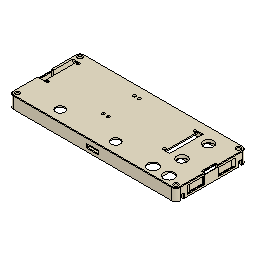
Font Plates (Autodesk Fusion 360 design; units mm, degrees)
Autodesk Fusion 360 part; units mm, degrees
sketch "Sketch1" plane through (0, 0, 0) normal (0, 0, 1) x (1, 0, 0)
  line L0 (0, 0) -> (200, 0)
  line L1 (200, 0) -> (200, 85)
  line L2 (200, 85) -> (0, 85)
  line L3 (0, 85) -> (0, 0)
  dimension "d1" = 200
  dimension "d2" = 85
  constraint horizontal L0
  constraint vertical L1
  constraint horizontal L2
  constraint vertical L3
  constraint coincident L0.start L3.end
  measures "d1" distance of L0.start L0.end
  measures "d2" distance of L0.start L2.end
extrude "Extrude1" add sketch "Sketch1" along normal blind 1.5 makes body 1
sketch "Sketch2" plane through (0, 0, 1.5) normal (0, 0, 1) x (-1, 0, 0)
  line L0 (0, -85) -> (0, 0)
  line L1 (0, 0) -> (-200, 0)
  line L2 (-200, 0) -> (-200, -85)
  line L3 (-200, -85) -> (0, -85)
  line L4 (-100, -85) -> (-100, 0) construction
  line L5 (0, -42.5) -> (-200, -42.5) construction
  line L6 (-3, -3) -> (-197, -3)
  line L7 (-197, -3) -> (-197, -82)
  line L8 (-197, -82) -> (-3, -82)
  line L9 (-3, -82) -> (-3, -3)
  dimension "d176" = -3
  constraint midpoint L1 L4.end
  constraint midpoint L0 L5.start
  constraint midpoint L3 L4.start
  constraint midpoint L2 L5.end
extrude "Extrude2" add sketch "Sketch2" along normal blind 13.7 bodies 1
sketch "Sketch4" plane through (197, 0, 0) normal (-1, 0, 0) x (0, -1, 0)
  line L0 (-50.25, 1.5) -> (-34.75, 1.5)
  line L1 (-34.75, 1.5) -> (-34.75, 9.1)
  line L2 (-34.75, 9.1) -> (-50.25, 9.1)
  line L3 (-50.25, 9.1) -> (-50.25, 1.5)
  line L4 (-42.5, 15.2) -> (-42.5, 1.5) construction
  line L5 (-82, 1.5) -> (-3, 1.5)
  line L6 (-3, 1.5) -> (-3, 15.2)
  line L7 (-3, 15.2) -> (-82, 15.2)
  line L8 (-82, 15.2) -> (-82, 1.5)
  dimension "d84" = 15.5
  dimension "d284" = 7.6
  constraint horizontal L0
  constraint vertical L1
  constraint horizontal L2
  constraint vertical L3
  constraint midpoint L0 L4.end
  constraint perpendicular L0 L4
  constraint coincident L4.end L5
  constraint midpoint L4.start L7
  measures "d84" distance of L1 L3
  measures "d284" distance of L0.end L1.end
extrude "Extrude4" cut sketch "Sketch4" against normal blind 1.85 contours L0 L1 L2 L3 L5 bodies 1
ref_plane "WorkPlane3" through (100, 42.5, 7.6) normal (-1, 0, 0) x (0, -1, 0)
mirror "Mirror1" about plane through (100, 42.5, 7.6) normal (-1, 0, 0) of "Extrude4"
sketch "Sketch6" plane through (0, 82, 0) normal (0, -1, 0) x (1, 0, 0)
  line L0 (93.5, 10.1) -> (106.5, 10.1)
  line L1 (106.5, 10.1) -> (106.5, 6.6)
  line L2 (106.5, 6.6) -> (93.5, 6.6)
  line L3 (93.5, 6.6) -> (93.5, 10.1)
  line L4 (100, 15.2) -> (100, 1.5) construction
  line L5 (100, 10.1) -> (100, 6.6) construction
  circle A0 centre (169, 8.35) radius 2
  line L6 (169, 15.2) -> (169, 1.5) construction
  circle A1 centre (31, 8.35) radius 2
  line L7 (3, 1.5) -> (197, 1.5)
  line L8 (197, 1.5) -> (197, 15.2)
  line L9 (197, 15.2) -> (3, 15.2)
  line L10 (3, 15.2) -> (3, 1.5)
  dimension "d25" = 13
  dimension "d26" = 3.5
  dimension "d27" = 4
  dimension "d179" = 28
  constraint horizontal L0
  constraint vertical L1
  constraint horizontal L2
  constraint vertical L3
  constraint midpoint L0 L5.start
  constraint midpoint L2 L5.end
  constraint midpoint L4 L5
  constraint midpoint A0.centre L6
  constraint symmetric L4 A0 A1
  constraint coincident L4.start L9
  constraint midpoint L4.start L9
  constraint midpoint L4.end L7
  constraint coincident L6.start L9
  constraint coincident L6.end L7
  measures "d25" distance of L0.start L0.end
  measures "d26" distance of L0.start L2.end
  measures "d27" diameter of A0
  measures "d179" distance of L6 L8
extrude "Extrude7" cut sketch "Sketch6" against normal through all and the other way through all contours L0 L1 L2 L3 bodies 1
sketch "Sketch3" plane through (0, 0, 0) normal (0, 0, -1) x (1, 0, 0)
  line L0 (0, 0) -> (0, -85)
  line L1 (0, -85) -> (200, -85)
  line L2 (200, -85) -> (200, 0)
  line L3 (200, 0) -> (0, 0)
  line L4 (200, -50.25) -> (197, -50.25)
  line L5 (197, -50.25) -> (197, -34.75)
  line L6 (197, -34.75) -> (200, -34.75)
  line L7 (200, -34.75) -> (200, -50.25)
  line L8 (100, -85) -> (100, 0) construction
  line L9 (3, -50.25) -> (3, -34.75)
  line L10 (3, -34.75) -> (0, -34.75)
  line L11 (0, -34.75) -> (0, -50.25)
  line L12 (0, -50.25) -> (3, -50.25)
  dimension "d11" = 3
  dimension "d12" = 15.5
  constraint horizontal L4
  constraint vertical L5
  constraint horizontal L6
  constraint vertical L7
  constraint coincident L2 L4.start
  constraint midpoint L2 L7
  constraint midpoint L1 L8.start
  constraint midpoint L3 L8.end
  constraint symmetric L4.start L8 L11.end
  constraint symmetric L4.end L8 L9.start
  constraint symmetric L5.end L8 L9.end
  constraint symmetric L6.end L8 L10.end
  measures "d11" distance of L4.start L4.end
  measures "d12" distance of L4.end L5.end
extrude "Extrude3" cut sketch "Sketch3" against normal blind 2.1 contours L0 L9 L10 L11 L12 | L2 L4 L5 L6 L7 bodies 1
sketch "Sketch25" plane through (200, 0, 0) normal (1, 0, 0) x (0, 1, 0)
  line L0 (34.75, 0) -> (34.75, 2.1)
  line L1 (34.75, 2.1) -> (50.25, 2.1)
  line L2 (50.25, 2.1) -> (50.25, 0)
  line L3 (50.25, 0) -> (85, 0)
  line L4 (85, 0) -> (85, 15.2)
  line L5 (85, 15.2) -> (0, 15.2)
  line L6 (0, 15.2) -> (0, 0)
  line L7 (0, 0) -> (34.75, 0)
  line L8 (42.5, 15.2) -> (42.5, 0) construction
  line L9 (78.9, 15.2) -> (75.9, 15.2)
  line L10 (75.9, 15.2) -> (75.9, 9.2)
  line L11 (75.9, 9.2) -> (78.9, 9.2)
  line L12 (78.9, 9.2) -> (78.9, 15.2)
  line L13 (77.4, 9.2) -> (77.4, 15.2) construction
  line L14 (9.1, 15.2) -> (9.1, 9.2)
  line L15 (9.1, 9.2) -> (6.1, 9.2)
  line L16 (6.1, 9.2) -> (6.1, 15.2)
  dimension "d248" = 3
  dimension "d249" = 6
  dimension "d250" = 34.9
  constraint midpoint L5 L8.start
  constraint perpendicular L5 L8
  constraint horizontal L9
  constraint vertical L10
  constraint horizontal L11
  constraint vertical L12
  constraint coincident L5 L9.start
  constraint midpoint L11 L13.start
  constraint midpoint L9 L13.end
  constraint symmetric L8 L9.start L16.end
  constraint symmetric L8 L9.end L14.start
  constraint symmetric L8 L10.end L14.end
  constraint symmetric L8 L11.end L15.end
  measures "d248" distance of L9.start L9.end
  measures "d249" distance of L9.start L11.end
  measures "d250" distance of L8 L13
extrude "Extrude28" cut sketch "Sketch25" against normal up to surface (3 mm away) contours L5 L14 L15 L16 | L5 L9 L10 L11 L12 bodies 1
sketch "Sketch26" plane through (200, 0, 0) normal (1, 0, 0) x (0, 1, 0)
  line L0 (78.9, 15.2) -> (78.9, 9.2)
  line L1 (78.9, 9.2) -> (75.9, 9.2)
  line L2 (75.9, 9.2) -> (75.9, 15.2)
  line L3 (75.9, 15.2) -> (9.1, 15.2)
  line L4 (9.1, 15.2) -> (9.1, 9.2)
  line L5 (9.1, 9.2) -> (6.1, 9.2)
  line L6 (6.1, 9.2) -> (6.1, 15.2)
  line L7 (6.1, 15.2) -> (0, 15.2)
  line L8 (0, 15.2) -> (0, 0)
  line L9 (0, 0) -> (34.75, 0)
  line L10 (34.75, 0) -> (34.75, 2.1)
  line L11 (34.75, 2.1) -> (50.25, 2.1)
  line L12 (50.25, 2.1) -> (50.25, 0)
  line L13 (50.25, 0) -> (85, 0)
  line L14 (85, 0) -> (85, 15.2)
  line L15 (85, 15.2) -> (78.9, 15.2)
  line L16 (67.5, 3.5) -> (51.5, 3.5)
  line L17 (51.5, 3.5) -> (51.5, 11.5)
  line L18 (51.5, 11.5) -> (67.5, 11.5)
  line L19 (67.5, 11.5) -> (67.5, 3.5)
  line L20 (67.5, 7.5) -> (51.5, 7.5) construction
  dimension "d253" = 16
  dimension "d254" = 8
  dimension "d255" = 17.5
  dimension "d256" = 7.5
  constraint horizontal L16
  constraint vertical L17
  constraint horizontal L18
  constraint vertical L19
  constraint midpoint L19 L20.start
  constraint midpoint L17 L20.end
  measures "d253" distance of L16.start L16.end
  measures "d254" distance of L16.start L18.end
  measures "d255" distance of L14 L19
  measures "d256" distance of L13 L20
extrude "Extrude29" cut sketch "Sketch26" against normal blind 1.5 contours L16 L17 L18 L19 bodies 1
sketch "Sketch28" plane through (0, 0, 3.5) normal (0, 0, 1) x (-1, 0, 0)
  line L0 (-200, -51.5) -> (-200, -67.5)
  line L1 (-200, -67.5) -> (-198.5, -67.5)
  line L2 (-198.5, -67.5) -> (-198.5, -51.5)
  line L3 (-198.5, -51.5) -> (-200, -51.5)
  line L4 (-200, -50.25) -> (-200, -85)
  line L5 (-198.5, -67.5) -> (-200, -71.1213)
  line L6 (-198.5, -67.5) -> (-194.5803, -67.5) construction
  dimension "d268" = 112.5
  constraint horizontal L6
  constraint coincident L1.end L2.start
  constraint coincident L4 L5.end
  measures "d268" angle of L5 L6
extrude "Extrude31" cut sketch "Sketch28" along normal up to surface (8 mm away) contours L1 L4 L5 bodies 1
ref_plane "WorkPlane5" through (100, 42.5, 7.6) normal (0, -1, 0) x (1, 0, 0)
mirror "Mirror5" about plane through (100, 42.5, 7.6) normal (0, -1, 0) of "Extrude29", "Extrude31"
mirror "Mirror4" about plane through (100, 42.5, 7.6) normal (-1, 0, 0) of "Extrude28", "Extrude29", "Extrude31", "Mirror5"
fillet "Fillet10" radius 5 8 edges at (0, 85, 7.6) (0, 0, 7.6) (200, 0, 7.6) (200, 85, 7.6) (197, 3, 8.35) (3, 3, 8.35) (3, 82, 8.35) (197, 82, 8.35) on bodies 1
chamfer "Chamfer9" distance 0.8 angle 45 4 faces at (69.3333, 84, 15.2) (69.3333, 1, 15.2) (199, 31.3667, 15.2) (1, 53.6333, 15.2) on bodies 1
chamfer "Chamfer7" distance 0.6 angle 45 16 edges at (100, 85, 0) (198.5355, 83.5355, 0) (200, 65.125, 0) (0, 65.125, 0) (1.4645, 83.5355, 0) (0, 19.875, 0) (1.4645, 1.4645, 0) (100, 0, 0) (198.5355, 1.4645, 0) (200, 19.875, 0) (197, 42.5, 0) (198.5, 50.25, 0) (198.5, 34.75, 0) (1.5, 50.25, 0) (3, 42.5, 0) (1.5, 34.75, 0) on bodies 1
chamfer "Chamfer8" distance 0.6 angle 45 50 edges at (100, 85, 10.1) (93.5, 85, 8.35) (100, 85, 6.6) (106.5, 85, 8.35) (1.15, 42.5, 2.1) (100, 0, 10.1) (106.5, 0, 8.35) (100, 0, 6.6) (93.5, 0, 8.35) (198.85, 42.5, 2.1) (200, 78.9, 11.8) (200, 75.9, 11.8) (196.9053, 77.9683, 9.2) (197, 76.45, 9.2) (196.6249, 78.9, 11.8) (197, 75.9, 11.8) (200, 77.4, 9.2) (200, 9.1, 11.8) (200, 7.6, 9.2) (197, 8.55, 9.2) (196.9053, 7.0317, 9.2) (197, 9.1, 11.8) (200, 6.1, 11.8) (196.6249, 6.1, 11.8) (3.0947, 7.0317, 9.2) (3, 8.55, 9.2) (3.3751, 6.1, 11.8) (0, 9.1, 11.8) (0, 7.6, 9.2) (0, 6.1, 11.8) (3, 9.1, 11.8) (3.3751, 78.9, 11.8) (3.0947, 77.9683, 9.2) (3, 76.45, 9.2) (3, 75.9, 11.8) (0, 75.9, 11.8) (0, 77.4, 9.2) (0, 78.9, 11.8) (0, 61.3107, 3.5) (0, 61.3107, 11.5) (0, 51.5, 7.5) (200, 61.3107, 3.5) (200, 51.5, 7.5) (200, 61.3107, 11.5) (0, 23.6893, 3.5) (0, 33.5, 7.5) (0, 23.6893, 11.5) (200, 23.6893, 11.5) (200, 33.5, 7.5) (200, 23.6893, 3.5) on bodies 1
sketch "Sketch13" plane through (0, 0, 0) normal (0, 0, 1) x (1, 0, 0)
  line L0 (5, 85) -> (195, 85)
  arc A0 (5, 85) -> (0, 80) centre (5, 80) ccw
  line L1 (0, 50.25) -> (0, 80)
  line L2 (0, 50.25) -> (0, 34.75)
  line L3 (0, 5) -> (0, 34.75)
  arc A1 (0, 5) -> (5, 0) centre (5, 5) ccw
  line L4 (195, 0) -> (5, 0)
  arc A2 (195, 0) -> (200, 5) centre (195, 5) ccw
  line L5 (200, 34.75) -> (200, 5)
  line L6 (200, 34.75) -> (200, 50.25)
  line L7 (200, 80) -> (200, 50.25)
  arc A3 (200, 80) -> (195, 85) centre (195, 80) ccw
  line L8 (200.1, 34.75) -> (200.1, 50.25)
  line L9 (200.1, 80) -> (200.1, 50.25)
  arc A4 (200.1, 80) -> (195, 85.1) centre (195, 80) ccw
  line L10 (5, 85.1) -> (195, 85.1)
  arc A5 (5, 85.1) -> (-0.1, 80) centre (5, 80) ccw
  line L11 (-0.1, 50.25) -> (-0.1, 80)
  line L12 (-0.1, 50.25) -> (-0.1, 34.75)
  line L13 (-0.1, 5) -> (-0.1, 34.75)
  arc A6 (-0.1, 5) -> (5, -0.1) centre (5, 5) ccw
  line L14 (195, -0.1) -> (5, -0.1)
  arc A7 (195, -0.1) -> (200.1, 5) centre (195, 5) ccw
  line L15 (200.1, 34.75) -> (200.1, 5)
  line L16 (-2.5, 5) -> (-2.5, 34.75)
  line L17 (-2.5, 50.25) -> (-2.5, 34.75)
  line L18 (-2.5, 50.25) -> (-2.5, 80)
  arc A8 (5, 87.5) -> (-2.5, 80) centre (5, 80) ccw
  line L19 (5, 87.5) -> (195, 87.5)
  arc A9 (202.5, 80) -> (195, 87.5) centre (195, 80) ccw
  line L20 (202.5, 80) -> (202.5, 50.25)
  line L21 (202.5, 34.75) -> (202.5, 50.25)
  line L22 (202.5, 34.75) -> (202.5, 5)
  arc A10 (195, -2.5) -> (202.5, 5) centre (195, 5) ccw
  line L23 (195, -2.5) -> (5, -2.5)
  arc A11 (-2.5, 5) -> (5, -2.5) centre (5, 5) ccw
  dimension "d191" = 0.1
  dimension "d192" = 2.5
extrude "Extrude14" add sketch "Sketch13" along normal mid plane 15.6 separate body contours L16 L17 L18 A8 L19 A9 L20 L21 L22 A10 L23 A11 makes body 2
sketch "Sketch12" plane through (0, 0, 0) normal (0, 0, -1) x (1, 0, 0)
  line L0 (3, -11.5) -> (8.5, -11.5)
  line L1 (8.5, -11.5) -> (8.5, -51.5)
  line L2 (8.5, -51.5) -> (3, -51.5)
  line L3 (3, -51.5) -> (3, -11.5)
  circle A0 centre (11, -13) radius 1.75
  circle A1 centre (78, -13) radius 1.75
  circle A2 centre (11, -50) radius 1.75
  circle A3 centre (78, -50) radius 1.75
  circle A4 centre (84, -13) radius 1.75
  circle A5 centre (151, -13) radius 1.75
  circle A6 centre (84, -50) radius 1.75
  circle A7 centre (151, -50) radius 1.75
  circle A8 centre (47.82, -71.5) radius 5.5
  circle A9 centre (114.18, -71.5) radius 5.5
  line L4 (153.5, -11.5) -> (159, -11.5)
  line L5 (159, -11.5) -> (159, -51.5)
  line L6 (159, -51.5) -> (153.5, -51.5)
  line L7 (153.5, -51.5) -> (153.5, -11.5)
  circle A10 centre (162.5, -75) radius 6.5
  circle A11 centre (181.5, -75) radius 6.5
  circle A12 centre (172, -18) radius 6.25
  circle A13 centre (172, -49.8) radius 6.25
  line L8 (162.5, -75) -> (181.5, -75) construction
  line L9 (172, -75) -> (172, 0) construction
  line L10 (200, -34.75) -> (200, -50.25)
  line L11 (200, -34.75) -> (200, -5)
  arc A14 (200, -5) -> (195, 0) centre (195, -5) ccw
  line L12 (195, 0) -> (5, 0)
  line L13 (200, -80) -> (200, -50.25)
  arc A15 (195, -85) -> (200, -80) centre (195, -80) ccw
  line L14 (5, -85) -> (195, -85)
  arc A16 (0, -80) -> (5, -85) centre (5, -80) ccw
  line L15 (0, -50.25) -> (0, -80)
  line L16 (0, -50.25) -> (0, -34.75)
  line L17 (0, -5) -> (0, -34.75)
  arc A17 (5, 0) -> (0, -5) centre (5, -5) ccw
  line L18 (23.32, -13) -> (72.32, -13)
  line L19 (72.32, -13) -> (72.32, -50)
  line L20 (72.32, -50) -> (23.32, -50)
  line L21 (23.32, -50) -> (23.32, -13)
  line L22 (47.82, -13) -> (47.82, -50) construction
  line L23 (78, -13) -> (78, -50) construction
  line L24 (72.32, -31.5) -> (78, -31.5) construction
  line L25 (89.68, -13) -> (138.68, -13)
  line L26 (138.68, -13) -> (138.68, -50)
  line L27 (138.68, -50) -> (89.68, -50)
  line L28 (89.68, -50) -> (89.68, -13)
  line L29 (114.18, -13) -> (114.18, -50) construction
  point P0 (72.32, -31.5)
  point P1 (78, -31.5)
  dimension "d97" = 5.5
  dimension "d100" = 40
  dimension "d102" = 3.5
  dimension "d109" = 67
  dimension "d110" = 67
  dimension "d111" = 11
  dimension "d115" = 5.5
  dimension "d116" = 40
  dimension "d118" = 13
  dimension "d121" = 19
  dimension "d193" = 13
  dimension "d194" = 11
  dimension "d195" = 37
  dimension "d196" = 6
  dimension "d197" = 11.5
  dimension "d198" = 3
  dimension "d200" = 71.5
  dimension "d201" = 153.5
  dimension "d202" = 172
  dimension "d205" = 75
  dimension "d278" = 18
  dimension "d279" = 31.8
  dimension "d283" = 12.5
  dimension "d285" = 49
  dimension "d286" = 37
  dimension "d287" = 36.82
  dimension "d298" = 49
  dimension "d299" = 37
  dimension "d328" = 36.82
  constraint horizontal L0
  constraint vertical L1
  constraint horizontal L2
  constraint vertical L3
  constraint equal A0 A2
  constraint equal A0 A1
  constraint equal A0 A3
  constraint horizontal A0.centre A1.centre
  constraint horizontal A2.centre A3.centre
  constraint vertical A0.centre A2.centre
  constraint vertical A1.centre A3.centre
  constraint equal A0 A4
  constraint equal A0 A5
  constraint equal A0 A6
  constraint equal A0 A7
  constraint horizontal A4.centre A5.centre
  constraint horizontal A1.centre A5.centre
  constraint horizontal A3.centre A6.centre
  constraint horizontal A6.centre A7.centre
  constraint vertical A4.centre A6.centre
  constraint vertical A5.centre A7.centre
  constraint equal A8 A9
  constraint horizontal A8.centre A9.centre
  constraint horizontal L4
  constraint vertical L5
  constraint horizontal L6
  constraint vertical L7
  constraint collinear L0 L4
  constraint equal A10 A11
  constraint horizontal A10.centre A11.centre
  constraint equal A12 A13
  constraint vertical A12.centre A13.centre
  constraint coincident A10.centre L8.start
  constraint coincident A11.centre L8.end
  constraint midpoint L8 L9.start
  constraint coincident A12.centre L9
  constraint horizontal L18
  constraint vertical L19
  constraint horizontal L20
  constraint vertical L21
  constraint midpoint L18 L22.start
  constraint midpoint L20 L22.end
  constraint coincident A1.centre L23.start
  constraint coincident A3.centre L23.end
  constraint midpoint L19 P0
  constraint midpoint L23 P1
  constraint horizontal P0 P1
  constraint coincident P0 L24.start
  constraint coincident P1 L24.end
  constraint horizontal L25
  constraint vertical L26
  constraint horizontal L27
  constraint vertical L28
  constraint midpoint L25 L29.start
  constraint midpoint L27 L29.end
  constraint collinear L18 L25
  constraint coincident A8.centre L22
  constraint coincident A9.centre L29
  measures "d97" distance of L0.start L0.end
  measures "d100" distance of L0.end L1.end
  measures "d102" diameter of A0
  measures "d109" distance of A4.centre A5.centre
  measures "d110" distance of A0.centre A1.centre
  measures "d111" diameter of A8
  measures "d115" distance of L4.start L4.end
  measures "d116" distance of L4.end L5.end
  measures "d118" diameter of A10
  measures "d121" distance of A10.centre A11.centre
  measures "d193" distance of A0.centre L12
  measures "d194" distance of A0.centre L17
  measures "d195" distance of A0.centre A2.centre
  measures "d196" distance of A1.centre A4.centre
  measures "d197" distance of L0 L12
  measures "d198" distance of L3 L17
  measures "d200" distance of A8.centre L12
  measures "d201" distance of L7 L17
  measures "d202" distance of L9 L16
  measures "d205" distance of A10.centre L12
  measures "d278" distance of A12.centre L12
  measures "d279" distance of A12.centre A13.centre
  measures "d283" diameter of A12
  measures "d285" distance of L18.start L18.end
  measures "d286" distance of L18.start L20.end
  measures "d287" distance of A0.centre L22
  measures "d298" distance of L25.start L25.end
  measures "d299" distance of L25.start L27.end
  measures "d328" distance of A5.centre L29
extrude "Extrude13" cut sketch "Sketch12" against normal through all contours L0 L1 L2 L3 | A0 | A1 | A2 | A3 | A4 | A5 | A6 | A7 | A8 | A9 | L4 L5 L6 L7 | A10 | A11 | A12 | A13 bodies 1
sketch "Sketch22" plane through (0, 0, 1.5) normal (0, 0, 1) x (-1, 0, 0)
  line L0 (-3, -51.5) -> (-8.5, -51.5)
  line L1 (-8.5, -51.5) -> (-8.5, -11.5)
  line L2 (-8.5, -11.5) -> (-3, -11.5)
  line L3 (-3, -11.5) -> (-3, -8)
  arc A0 (-3, -8) -> (-8, -3) centre (-8, -8) ccw
  line L4 (-8, -3) -> (-192, -3)
  arc A1 (-192, -3) -> (-197, -8) centre (-192, -8) ccw
  line L5 (-197, -8) -> (-197, -34.75)
  line L6 (-197, -34.75) -> (-197, -50.25)
  arc A2 (-197, -77) -> (-192, -82) centre (-192, -77) ccw
  line L7 (-192, -82) -> (-8, -82)
  arc A3 (-8, -82) -> (-3, -77) centre (-8, -77) ccw
  line L8 (-3, -77) -> (-3, -51.5)
  circle A4 centre (-11, -13) radius 1.75
  circle A5 centre (-84, -13) radius 1.75
  circle A6 centre (-114.18, -71.5) radius 5.5
  circle A7 centre (-172, -18) radius 6.25
  circle A8 centre (-181.5, -75) radius 6.5
  line L9 (-153.5, -11.5) -> (-153.5, -51.5)
  line L10 (-153.5, -51.5) -> (-159, -51.5)
  line L11 (-159, -51.5) -> (-159, -11.5)
  line L12 (-159, -11.5) -> (-153.5, -11.5)
  circle A9 centre (-84, -50) radius 1.75
  circle A10 centre (-47.82, -71.5) radius 5.5
  circle A11 centre (-78, -13) radius 1.75
  circle A12 centre (-151, -50) radius 1.75
  circle A13 centre (-172, -49.8) radius 6.25
  circle A14 centre (-162.5, -75) radius 6.5
  circle A15 centre (-151, -13) radius 1.75
  circle A16 centre (-78, -50) radius 1.75
  circle A17 centre (-11, -50) radius 1.75
  line L13 (-163.1, -10.6) -> (-180.9, -10.6)
  line L14 (-180.9, -10.6) -> (-180.9, -25.4)
  line L15 (-180.9, -25.4) -> (-163.1, -25.4)
  line L16 (-163.1, -25.4) -> (-163.1, -10.6)
  line L17 (-163.1, -10.6) -> (-180.9, -25.4) construction
  line L18 (-180.9, -10.6) -> (-163.1, -25.4) construction
  line L19 (-160.1, -7.6) -> (-183.9, -7.6)
  line L20 (-183.9, -7.6) -> (-183.9, -28.4)
  line L21 (-183.9, -28.4) -> (-160.1, -28.4)
  line L22 (-160.1, -28.4) -> (-160.1, -7.6)
  line L23 (-160.1, -7.6) -> (-183.9, -28.4) construction
  line L24 (-183.9, -7.6) -> (-160.1, -28.4) construction
  line L25 (-163.1, -42.4) -> (-180.9, -42.4)
  line L26 (-180.9, -42.4) -> (-180.9, -57.2)
  line L27 (-180.9, -57.2) -> (-163.1, -57.2)
  line L28 (-163.1, -57.2) -> (-163.1, -42.4)
  line L29 (-163.1, -42.4) -> (-180.9, -57.2) construction
  line L30 (-180.9, -42.4) -> (-163.1, -57.2) construction
  line L31 (-160.1, -39.4) -> (-183.9, -39.4)
  line L32 (-183.9, -39.4) -> (-183.9, -60.2)
  line L33 (-183.9, -60.2) -> (-160.1, -60.2)
  line L34 (-160.1, -60.2) -> (-160.1, -39.4)
  line L35 (-160.1, -39.4) -> (-183.9, -60.2) construction
  line L36 (-183.9, -39.4) -> (-160.1, -60.2) construction
  line L37 (-197, -50.25) -> (-197, -77)
  point P0 (-172, -18)
  point P1 (-172, -18)
  point P2 (-172, -49.8)
  point P3 (-172, -49.8)
  dimension "d230" = 14.8
  dimension "d231" = 17.8
  dimension "d232" = 3
  dimension "d233" = 3
  constraint horizontal L13
  constraint perpendicular L13 L14
  constraint parallel L13 L15
  constraint parallel L14 L16
  constraint coincident L17 P1
  constraint coincident L18 P1
  constraint coincident P1 P0
  constraint horizontal L19
  constraint perpendicular L19 L20
  constraint parallel L19 L21
  constraint parallel L20 L22
  constraint coincident L23 P1
  constraint coincident L24 P1
  constraint horizontal L25
  constraint perpendicular L25 L26
  constraint parallel L25 L27
  constraint parallel L26 L28
  constraint coincident L29 P3
  constraint coincident L30 P3
  constraint coincident P3 P2
  constraint horizontal L31
  constraint perpendicular L31 L32
  constraint parallel L31 L33
  constraint parallel L32 L34
  constraint coincident L35 P3
  constraint coincident L36 P3
  constraint equal L19 L31
  constraint equal L13 L25
  constraint equal L16 L28
  constraint equal L22 L34
  measures "d230" distance of L13.start L15.end
  measures "d231" distance of L13.start L13.end
  measures "d232" distance of L16 L22
  measures "d233" distance of L13 L19
extrude "Extrude23" add sketch "Sketch22" along normal blind 3 contours L13 L14 L15 L16 | L25 L26 L27 L28 bodies 1
extrude "Extrude24" add sketch "Sketch22" along normal blind 6 contours L19 L20 L21 L22 | L31 L32 L33 L34 bodies 1
chamfer "Chamfer10" distance 1 angle 45 2 edges at (177.827, 47.5399, 4.5) (177.827, 15.7399, 4.5) on bodies 1
sketch "Sketch24" plane through (0, 0, 1.5) normal (0, 0, 1) x (-1, 0, 0)
  line L0 (-160.1, -28.4) -> (-183.9, -28.4)
  line L1 (-183.9, -28.4) -> (-183.9, -7.6)
  line L2 (-183.9, -7.6) -> (-160.1, -7.6)
  line L3 (-160.1, -7.6) -> (-160.1, -28.4)
  line L4 (-160.1, -60.2) -> (-183.9, -60.2)
  line L5 (-183.9, -60.2) -> (-183.9, -39.4)
  line L6 (-183.9, -39.4) -> (-160.1, -39.4)
  line L7 (-160.1, -39.4) -> (-160.1, -60.2)
  line L8 (-3, -51.5) -> (-8.5, -51.5)
  line L9 (-8.5, -51.5) -> (-8.5, -11.5)
  line L10 (-8.5, -11.5) -> (-3, -11.5)
  line L11 (-3, -11.5) -> (-3, -8)
  arc A0 (-3, -8) -> (-8, -3) centre (-8, -8) ccw
  line L12 (-8, -3) -> (-192, -3)
  arc A1 (-192, -3) -> (-197, -8) centre (-192, -8) ccw
  line L13 (-197, -8) -> (-197, -34.75)
  line L14 (-197, -34.75) -> (-197, -50.25)
  arc A2 (-197, -77) -> (-192, -82) centre (-192, -77) ccw
  line L15 (-192, -82) -> (-8, -82)
  arc A3 (-8, -82) -> (-3, -77) centre (-8, -77) ccw
  line L16 (-3, -77) -> (-3, -51.5)
  circle A4 centre (-11, -13) radius 1.75
  circle A5 centre (-84, -13) radius 1.75
  circle A6 centre (-114.18, -71.5) radius 5.5
  circle A7 centre (-181.5, -75) radius 6.5
  line L17 (-153.5, -11.5) -> (-153.5, -51.5)
  line L18 (-153.5, -51.5) -> (-159, -51.5)
  line L19 (-159, -51.5) -> (-159, -11.5)
  line L20 (-159, -11.5) -> (-153.5, -11.5)
  circle A8 centre (-84, -50) radius 1.75
  circle A9 centre (-47.82, -71.5) radius 5.5
  circle A10 centre (-78, -13) radius 1.75
  circle A11 centre (-151, -50) radius 1.75
  circle A12 centre (-162.5, -75) radius 6.5
  circle A13 centre (-151, -13) radius 1.75
  circle A14 centre (-78, -50) radius 1.75
  circle A15 centre (-11, -50) radius 1.75
  line L21 (-175, -3) -> (-169, -3)
  line L22 (-169, -3) -> (-169, -82)
  line L23 (-169, -82) -> (-175, -82)
  line L24 (-175, -82) -> (-175, -3)
  line L25 (-172, -82) -> (-172, -3) construction
  line L26 (-181.5, -75) -> (-162.5, -75) construction
  line L27 (-197, -50.25) -> (-197, -77)
  point P0 (-172, -75)
  constraint horizontal L21
  constraint vertical L22
  constraint horizontal L23
  constraint vertical L24
  constraint coincident L15 L22.end
  constraint coincident L12 L21.start
  constraint midpoint L23 L25.start
  constraint midpoint L21 L25.end
  constraint tangent A12 L22
  constraint coincident A7.centre L26.start
  constraint coincident A12.centre L26.end
  constraint midpoint L26 P0
  constraint coincident L25 P0
extrude "Extrude26" add sketch "Sketch24" along normal blind 6 contours L0 L6 L22 L24 | L2 L12 L21 L22 L24 bodies 1
extrude "Extrude27" add sketch "Sketch24" along normal blind 2 contours L4 L15 L22 L23 L24 bodies 1
chamfer "Chamfer11" distance 2 angle 45 12 edges at (88.5, 3, 1.5) (4.4645, 4.4645, 1.5) (3, 9.75, 1.5) (183.5, 3, 1.5) (195.5355, 4.4645, 1.5) (197, 21.375, 1.5) (3, 64.25, 1.5) (88.5, 82, 1.5) (4.4645, 80.5355, 1.5) (183.5, 82, 1.5) (197, 63.625, 1.5) (195.5355, 80.5355, 1.5) on bodies 1
chamfer "Chamfer12" distance 2 angle 45 8 edges at (169, 33.9, 1.5) (169, 5.3, 1.5) (169, 67.6, 1.5) (175, 67.6, 1.5) (175, 33.9, 1.5) (175, 5.3, 1.5) (175, 78.5, 1.5) (169, 78.5, 1.5) on bodies 1
sketch "Sketch23" plane through (0, 0, 1.5) normal (0, 0, 1) x (-1, 0, 0)
  line L0 (-5, -77) -> (-5, -51.5)
  line L1 (-5, -51.5) -> (-8.5, -51.5)
  line L2 (-8.5, -51.5) -> (-8.5, -11.5)
  line L3 (-8.5, -11.5) -> (-5, -11.5)
  line L4 (-5, -11.5) -> (-5, -8)
  arc A0 (-5, -8) -> (-8, -5) centre (-8, -8) ccw
  line L5 (-8, -5) -> (-167, -5)
  arc A1 (-158.3467, -80) -> (-167, -70.3096) centre (-162.5, -75) ccw
  line L6 (-158.3467, -80) -> (-8, -80)
  arc A2 (-8, -80) -> (-5, -77) centre (-8, -77) ccw
  line L7 (-160.1, -28.4) -> (-167, -28.4)
  line L8 (-167, -7.6) -> (-160.1, -7.6)
  line L9 (-160.1, -7.6) -> (-160.1, -28.4)
  line L10 (-160.1, -60.2) -> (-167, -60.2)
  line L11 (-167, -39.4) -> (-160.1, -39.4)
  line L12 (-160.1, -39.4) -> (-160.1, -60.2)
  circle A3 centre (-11, -13) radius 1.75
  circle A4 centre (-84, -13) radius 1.75
  circle A5 centre (-114.18, -71.5) radius 5.5
  line L13 (-153.5, -11.5) -> (-153.5, -51.5)
  line L14 (-153.5, -51.5) -> (-159, -51.5)
  line L15 (-159, -51.5) -> (-159, -11.5)
  line L16 (-159, -11.5) -> (-153.5, -11.5)
  circle A6 centre (-84, -50) radius 1.75
  circle A7 centre (-47.82, -71.5) radius 5.5
  circle A8 centre (-78, -13) radius 1.75
  circle A9 centre (-151, -50) radius 1.75
  circle A10 centre (-151, -13) radius 1.75
  circle A11 centre (-78, -50) radius 1.75
  circle A12 centre (-11, -50) radius 1.75
  circle A13 centre (-114.18, -71.5) radius 11.5
  circle A14 centre (-47.82, -71.5) radius 11.5
  line L17 (-167, -60.2) -> (-167, -70.3096)
  line L18 (-167, -5) -> (-167, -7.6)
  line L19 (-167, -28.4) -> (-167, -39.4)
  dimension "d240" = 23
  constraint concentric A5 A13
  constraint concentric A7 A14
  constraint equal A13 A14
  measures "d240" diameter of A13
extrude "Extrude25" cut sketch "Sketch23" along normal up to surface (13.7 mm away) contours L6 A14 | L6 A13 picked at (-45.6834, -80.3493) picked at (-112.0434, -80.3493) bodies 1
sketch "Sketch14" plane through (0, 0, -7.8) normal (0, 0, -1) x (1, 0, 0)
  line L0 (-5.5, -5) -> (-5.5, -80)
  arc A0 (-5.5, -80) -> (5, -90.5) centre (5, -80) ccw
  line L1 (5, -90.5) -> (195, -90.5)
  arc A1 (195, -90.5) -> (205.5, -80) centre (195, -80) ccw
  line L2 (205.5, -80) -> (205.5, -5)
  arc A2 (205.5, -5) -> (195, 5.5) centre (195, -5) ccw
  line L3 (195, 5.5) -> (5, 5.5)
  arc A3 (5, 5.5) -> (-5.5, -5) centre (5, -5) ccw
  arc A4 (195, -85.1) -> (200.1, -80) centre (195, -80) ccw
  line L4 (195, -85.1) -> (5, -85.1)
  arc A5 (-0.1, -80) -> (5, -85.1) centre (5, -80) ccw
  line L5 (-0.1, -80) -> (-0.1, -5)
  arc A6 (5, 0.1) -> (-0.1, -5) centre (5, -5) ccw
  line L6 (5, 0.1) -> (195, 0.1)
  arc A7 (200.1, -5) -> (195, 0.1) centre (195, -5) ccw
  line L7 (200.1, -5) -> (200.1, -80)
  line L8 (-2.5, -5) -> (-2.5, -80)
  arc A8 (-2.5, -80) -> (5, -87.5) centre (5, -80) ccw
  line L9 (5, -87.5) -> (195, -87.5)
  arc A9 (195, -87.5) -> (202.5, -80) centre (195, -80) ccw
  line L10 (202.5, -80) -> (202.5, -5)
  arc A10 (202.5, -5) -> (195, 2.5) centre (195, -5) ccw
  line L11 (195, 2.5) -> (5, 2.5)
  arc A11 (5, 2.5) -> (-2.5, -5) centre (5, -5) ccw
  constraint tangent A2 L3
  constraint tangent L2 A2
  constraint tangent A0 L1
  constraint tangent A1 L2
  constraint tangent L1 A1
  constraint tangent L0 A0
  constraint tangent L3 A3
  constraint tangent L0 A3
extrude "Extrude15" add sketch "Sketch14" along normal blind 2.5 separate body contours L0 A0 L1 A1 L2 A2 L3 A3 | A4 L4 A5 L5 A6 L6 A7 L7 | L8 A8 L9 A9 L10 A10 L11 A11 makes body 3
sketch "Sketch15" plane through (0, 0, -10.3) normal (0, 0, -1) x (1, 0, 0)
  arc A0 (5, 5.5) -> (-5.5, -5) centre (5, -5) ccw
  line L0 (-5.5, -5) -> (-5.5, -80)
  arc A1 (-5.5, -80) -> (5, -90.5) centre (5, -80) ccw
  line L1 (5, -90.5) -> (195, -90.5)
  arc A2 (195, -90.5) -> (205.5, -80) centre (195, -80) ccw
  line L2 (205.5, -80) -> (205.5, -5)
  arc A3 (205.5, -5) -> (195, 5.5) centre (195, -5) ccw
  line L3 (195, 5.5) -> (5, 5.5)
  circle A4 centre (172, -18) radius 6.25 construction
  circle A5 centre (172, -49.8) radius 6.25 construction
  circle A6 centre (181.5, -75) radius 6.5
  circle A7 centre (162.5, -75) radius 6.5
  circle A8 centre (114.18, -71.5) radius 5.5 construction
  circle A9 centre (47.82, -71.5) radius 5.5 construction
  line L4 (169.75, -21.25) -> (174.25, -21.25)
  arc A10 (174.25, -21.25) -> (174.25, -14.75) centre (174.25, -18) ccw
  line L5 (174.25, -14.75) -> (169.75, -14.75)
  arc A11 (169.75, -14.75) -> (169.75, -21.25) centre (169.75, -18) ccw
  line L6 (165.75, -18) -> (178.25, -18) construction
  line L7 (169.75, -53.05) -> (174.25, -53.05)
  arc A12 (174.25, -53.05) -> (174.25, -46.55) centre (174.25, -49.8) ccw
  line L8 (174.25, -46.55) -> (169.75, -46.55)
  arc A13 (169.75, -46.55) -> (169.75, -53.05) centre (169.75, -49.8) ccw
  line L9 (169.75, -49.8) -> (174.25, -49.8) construction
  circle A14 centre (114.18, -71.5) radius 15.75
  circle A15 centre (47.82, -71.5) radius 15.75
  line L10 (174.25, -18) -> (169.75, -18) construction
  line L11 (47.82, -87.25) -> (47.82, 5.5) construction
  line L12 (114.18, -87.25) -> (114.18, 11) construction
  line L13 (23.32, -50) -> (23.32, -13)
  line L14 (23.32, -13) -> (72.32, -13)
  line L15 (72.32, -13) -> (72.32, -50)
  line L16 (72.32, -50) -> (23.32, -50)
  line L17 (89.68, -50) -> (89.68, -13)
  line L18 (89.68, -13) -> (138.68, -13)
  line L19 (138.68, -13) -> (138.68, -50)
  line L20 (138.68, -50) -> (89.68, -50)
  point P0 (172, -18)
  point P1 (172, -49.8)
  dimension "d165" = 6.5
  dimension "d166" = 31.5
  dimension "d174" = 4.5
  constraint tangent L4 A10
  constraint tangent A10 L5
  constraint parallel L4 L5
  constraint tangent L5 A11
  constraint tangent L4 A11
  constraint coincident A4 L6.end
  constraint horizontal L6
  constraint coincident P0 A4.centre
  constraint midpoint L6 P0
  constraint tangent L7 A12
  constraint tangent A12 L8
  constraint parallel L7 L8
  constraint tangent L8 A13
  constraint tangent L7 A13
  constraint horizontal L9
  constraint coincident P1 A5.centre
  constraint midpoint L9 P1
  constraint equal L5 L8
  constraint equal A10 A12
  constraint concentric A8 A14
  constraint concentric A9 A15
  constraint equal A14 A15
  constraint coincident A10.centre L10.start
  constraint coincident A11.centre L10.end
  constraint midpoint L6 L10
  constraint coincident L6 A10.centre
  constraint coincident A15 L11.start
  constraint coincident L3 L11.end
  constraint perpendicular L3 L11
  constraint coincident A9.centre L11
  constraint coincident A14 L12.start
  constraint perpendicular L3 L12
  constraint coincident A8.centre L12
  measures "d165" diameter of A10
  measures "d166" diameter of A14
  measures "d174" distance of A11.centre A10.centre
extrude "Extrude17" cut sketch "Sketch15" against normal up to surface (2.5 mm away) contours A6 | A7 | L4 A10 L5 A11 | L7 A12 L8 A13 | A14 | A15 | L13 L14 L15 L16 | L17 L18 L19 L20 bodies 3
sketch "Sketch20" plane through (0, 0, -10.3) normal (0, 0, -1) x (1, 0, 0)
  line L0 (169.75, -14.75) -> (174.25, -14.75)
  arc A0 (174.25, -21.25) -> (174.25, -14.75) centre (174.25, -18) ccw
  line L1 (174.25, -21.25) -> (169.75, -21.25)
  arc A1 (169.75, -14.75) -> (169.75, -21.25) centre (169.75, -18) ccw
  circle A2 centre (47.82, -71.5) radius 15.75
  circle A3 centre (162.5, -75) radius 6.5
  line L2 (169.75, -46.55) -> (174.25, -46.55)
  arc A4 (174.25, -53.05) -> (174.25, -46.55) centre (174.25, -49.8) ccw
  line L3 (174.25, -53.05) -> (169.75, -53.05)
  arc A5 (169.75, -46.55) -> (169.75, -53.05) centre (169.75, -49.8) ccw
  circle A6 centre (114.18, -71.5) radius 15.75
  circle A7 centre (181.5, -75) radius 6.5
  arc A8 (5, 5.5) -> (-5.5, -5) centre (5, -5) ccw
  line L4 (-5.5, -5) -> (-5.5, -80)
  arc A9 (-5.5, -80) -> (5, -90.5) centre (5, -80) ccw
  line L5 (5, -90.5) -> (195, -90.5)
  arc A10 (195, -90.5) -> (205.5, -80) centre (195, -80) ccw
  line L6 (205.5, -80) -> (205.5, -5)
  arc A11 (205.5, -5) -> (195, 5.5) centre (195, -5) ccw
  line L7 (195, 5.5) -> (5, 5.5)
  arc A12 (5, 0) -> (0, -5) centre (5, -5) ccw
  arc A13 (200, -5) -> (195, 0) centre (195, -5) ccw
  arc A14 (195, -85) -> (200, -80) centre (195, -80) ccw
  arc A15 (0, -80) -> (5, -85) centre (5, -80) ccw
  circle A16 centre (5, -5) radius 1.6
  circle A17 centre (195, -5) radius 1.6
  circle A18 centre (195, -80) radius 1.6
  circle A19 centre (5, -80) radius 1.6
  line L8 (72.32, -50) -> (23.32, -50)
  line L9 (23.32, -50) -> (23.32, -13)
  line L10 (23.32, -13) -> (72.32, -13)
  line L11 (72.32, -13) -> (72.32, -50)
  line L12 (138.68, -50) -> (89.68, -50)
  line L13 (89.68, -50) -> (89.68, -13)
  line L14 (89.68, -13) -> (138.68, -13)
  line L15 (138.68, -13) -> (138.68, -50)
  dimension "d206" = 3.2
  constraint concentric A12 A16
  constraint concentric A13 A17
  constraint concentric A14 A18
  constraint concentric A15 A19
  constraint equal A16 A17
  constraint equal A16 A18
  constraint equal A16 A19
  measures "d206" diameter of A16
extrude "Extrude20" cut sketch "Sketch20" against normal up to surface (2.5 mm away) contours A16 | A17 | A18 | A19 bodies 3
sketch "Sketch21" plane through (0, 0, 0) normal (0, 0, -1) x (1, 0, 0)
  line L0 (3, -34.15) -> (3, -11.5)
  line L1 (3, -11.5) -> (8.5, -11.5)
  line L2 (8.5, -11.5) -> (8.5, -51.5)
  line L3 (8.5, -51.5) -> (3, -51.5)
  line L4 (3, -51.5) -> (3, -50.85)
  line L5 (3, -50.85) -> (0.6, -50.85)
  line L6 (0.6, -50.85) -> (0.6, -80)
  arc A0 (0.6, -80) -> (5, -84.4) centre (5, -80) ccw
  line L7 (5, -84.4) -> (195, -84.4)
  arc A1 (195, -84.4) -> (199.4, -80) centre (195, -80) ccw
  line L8 (199.4, -80) -> (199.4, -50.85)
  line L9 (199.4, -50.85) -> (196.4, -50.85)
  line L10 (196.4, -50.85) -> (196.4, -34.15)
  line L11 (196.4, -34.15) -> (199.4, -34.15)
  line L12 (199.4, -34.15) -> (199.4, -5)
  arc A2 (199.4, -5) -> (195, -0.6) centre (195, -5) ccw
  line L13 (195, -0.6) -> (5, -0.6)
  arc A3 (5, -0.6) -> (0.6, -5) centre (5, -5) ccw
  line L14 (0.6, -5) -> (0.6, -34.15)
  line L15 (0.6, -34.15) -> (3, -34.15)
  circle A4 centre (11, -13) radius 1.75
  circle A5 centre (84, -13) radius 1.75
  circle A6 centre (114.18, -71.5) radius 5.5
  circle A7 centre (172, -18) radius 6.25
  circle A8 centre (181.5, -75) radius 6.5
  line L16 (153.5, -51.5) -> (153.5, -11.5)
  line L17 (153.5, -11.5) -> (159, -11.5)
  line L18 (159, -11.5) -> (159, -51.5)
  line L19 (159, -51.5) -> (153.5, -51.5)
  circle A9 centre (84, -50) radius 1.75
  circle A10 centre (47.82, -71.5) radius 5.5
  circle A11 centre (78, -13) radius 1.75
  circle A12 centre (151, -50) radius 1.75
  circle A13 centre (172, -49.8) radius 6.25
  circle A14 centre (162.5, -75) radius 6.5
  circle A15 centre (151, -13) radius 1.75
  circle A16 centre (78, -50) radius 1.75
  circle A17 centre (11, -50) radius 1.75
  circle A18 centre (5, -5) radius 2
  circle A19 centre (5, -5) radius 4
  circle A20 centre (195, -5) radius 2
  circle A21 centre (195, -5) radius 4
  circle A22 centre (195, -80) radius 2
  circle A23 centre (195, -80) radius 4
  circle A24 centre (5, -80) radius 2
  circle A25 centre (5, -80) radius 4
  circle A26 centre (5, -5) radius 1.6
  circle A27 centre (5, -80) radius 1.6
  circle A28 centre (195, -80) radius 1.6
  circle A29 centre (195, -5) radius 1.6
  dimension "d209" = 4
  dimension "d224" = 2
  constraint concentric A20 A21
  constraint concentric A22 A23
  constraint equal A18 A20
  constraint equal A19 A21
  constraint equal A18 A22
  constraint equal A19 A23
  constraint equal A18 A24
  constraint equal A19 A25
  constraint concentric A18 A26
  constraint concentric A20 A29
  constraint concentric A22 A28
  constraint concentric A24 A27
  constraint concentric A24 A25
  measures "d209" diameter of A18
  measures "d224" distance of A18 A19
extrude "Extrude21" cut sketch "Sketch21" against normal up to surface (15.2 mm away) contours A18 | A20 | A22 | A24 | A26 | A27 | A28 | A29 bodies 1
extrude "Extrude22" add sketch "Sketch21" against normal up to surface (9.2 mm away) contours A19 | A21 | A23 | A25 bodies 1
chamfer "Chamfer14" distance 0.8 angle 45 4 edges at (193.1353, 79.2768, 0) (193.1353, 4.2768, 0) (3.1353, 4.2768, 0) (3.1353, 79.2768, 0) on bodies 1
move_body "Move1" bodies 3 2 1 to x (-1, 0, 0) y (0, 1, 0) z (0, 0, -1) at (0, 0, 0)
move_body "Move2" bodies 1 3 2 to x (-1, 0, 0) y (0, -1, 0) z (0, 0, 1) at (0, 0, 0)
move_body "Move3" bodies 3 2 1 to x (1, 0, 0) y (0, 1, 0) z (0, 0, 1) at (0, 90.5, 0)
sketch "Export" plane through (0, 0, 0) normal (0, 0, 1) x (1, 0, 0)
  circle A0 centre (5, 85.5) radius 1.6
  circle A1 centre (195, 85.5) radius 1.6
  circle A2 centre (5, 10.5) radius 1.6
  circle A3 centre (195, 10.5) radius 1.6
  circle A4 centre (47.82, 19) radius 15.75
  circle A5 centre (162.5, 15.5) radius 6.5
  line L0 (169.75, 43.95) -> (174.25, 43.95)
  arc A6 (174.25, 37.45) -> (174.25, 43.95) centre (174.25, 40.7) ccw
  line L1 (174.25, 37.45) -> (169.75, 37.45)
  arc A7 (169.75, 43.95) -> (169.75, 37.45) centre (169.75, 40.7) ccw
  circle A8 centre (114.18, 19) radius 15.75
  circle A9 centre (181.5, 15.5) radius 6.5
  arc A10 (5, 96) -> (-5.5, 85.5) centre (5, 85.5) ccw
  line L2 (-5.5, 85.5) -> (-5.5, 10.5)
  arc A11 (-5.5, 10.5) -> (5, 0) centre (5, 10.5) ccw
  line L3 (5, 0) -> (195, 0)
  arc A12 (195, 0) -> (205.5, 10.5) centre (195, 10.5) ccw
  line L4 (205.5, 10.5) -> (205.5, 85.5)
  arc A13 (205.5, 85.5) -> (195, 96) centre (195, 85.5) ccw
  line L5 (195, 96) -> (5, 96)
  line L6 (72.32, 40.5) -> (23.32, 40.5)
  line L7 (23.32, 40.5) -> (23.32, 77.5)
  line L8 (23.32, 77.5) -> (72.32, 77.5)
  line L9 (72.32, 77.5) -> (72.32, 40.5)
  line L10 (138.68, 40.5) -> (89.68, 40.5)
  line L11 (89.68, 40.5) -> (89.68, 77.5)
  line L12 (89.68, 77.5) -> (138.68, 77.5)
  line L13 (138.68, 77.5) -> (138.68, 40.5)
  arc A14 (169.75, 75.75) -> (169.75, 69.25) centre (169.75, 72.5) ccw
  line L14 (169.75, 75.75) -> (174.25, 75.75)
  arc A15 (174.25, 69.25) -> (174.25, 75.75) centre (174.25, 72.5) ccw
  line L15 (174.25, 69.25) -> (169.75, 69.25)
chamfer "Chamfer13" distance 1 angle 45 8 edges at (205.5, 48, 10.3) (202.4246, 92.9246, 10.3) (100, 96, 10.3) (-2.4246, 92.9246, 10.3) (-5.5, 48, 10.3) (-2.4246, 3.0754, 10.3) (100, 0, 10.3) (202.4246, 3.0754, 10.3) measured on face at (4.1067, 45.5, 10.3) measured on face at (4.1067, 45.5, 10.3) measured on face at (4.1067, 45.5, 10.3) measured on face at (4.1067, 45.5, 10.3) measured on face at (4.1067, 45.5, 10.3) measured on face at (4.1067, 45.5, 10.3) measured on face at (4.1067, 45.5, 10.3) measured on face at (4.1067, 45.5, 10.3) on bodies 3
hidden bodies 2 3
equation "d9 = Backplate_Lip_Height - Backplate_Thickness"
equation "d16 = -3 mm + 1.15 mm"
equation "HS_Clearance = 2 mm"
equation "d109 = 151 mm - 84 mm"
equation "d110 = 78 mm - 11 mm"
equation "d121 = 181.5 mm - 162.5 mm"
equation "Backplate_Lip_Height = 15.2 mm"
equation "Backplate_Thickness = 1.5 mm"
equation "d255 = 33.5 mm - 16 mm"
equation "d268 = 22.5 deg + 90 deg"
